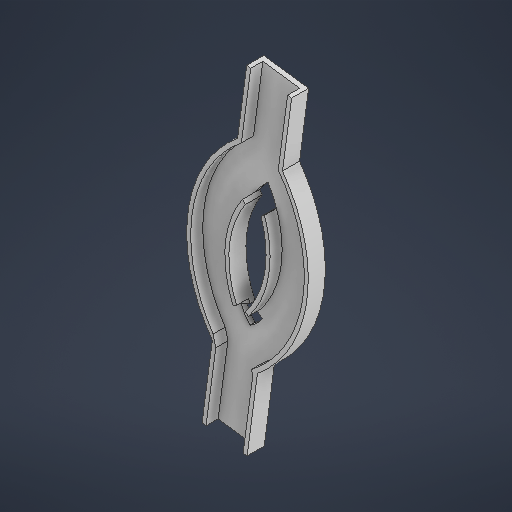
# Autodesk Inventor part: outside3
Saved by Autodesk Inventor 2026.2 (Build 302298000, 298)
## iProperties
Created: 2026-03-14
Part Number: outside3
Material: Generic
Document SubType Name: Modeling
Designer: danda
Density: 1 g/cm^3
Appearance: Default
Author: danda
Autodesk Inventor part; units mm, degrees
ref_plane "YZ Plane" through (0, 0, 0) normal (1, 0, 0) x (0, 1, 0)
ref_plane "XZ Plane" through (0, 0, 0) normal (0, 1, 0) x (-1, 0, 0)
ref_plane "XY Plane" through (0, 0, 0) normal (0, 0, 1) x (1, 0, 0)
sketch "Sketch1" plane through (0, 0, 0) normal (0, 0, 1) x (1, 0, 0)
  arc A0 (967.6192, 924.0732) -> (967.7873, 1075.2272) centre (902.2196, 999.723) ccw
  arc A1 (983.2683, 893.0126) -> (983.4428, 1106.3006) centre (902.2196, 999.723) ccw
  line L0 (965.7611, 927.7614) -> (985.0977, 889.3816)
  line L1 (966.6908, 925.9161) -> (1011.6908, 925.9161) construction
  arc A2 (985.0977, 889.3816) -> (985.2727, 1109.9327) centre (902.2196, 999.723) ccw
  line L2 (965.9281, 1071.5369) -> (985.2727, 1109.9327)
  arc A3 (965.7611, 927.7614) -> (965.9281, 1071.5369) centre (902.2196, 999.723) ccw
  line L3 (977.4986, 940.149) -> (980.6353, 937.6667)
  point P0 (0, 0)
  point P1 (983.9681, 893.1)
  point P2 (990.6031, 1100.4422)
  point P3 (968.1775, 1074.8866)
  dimension "d28" = 100
  dimension "d33" = 63.26
  dimension "d34" = 4
  dimension "d40" = 4
  dimension "d41" = 4
  constraints: 10 point on circle, 8 end point, 5 point on line, 4 centre point, 1 horizontal
  measures "d28" radius of A0
  measures "d33" angle of L0 L1
  measures "d34" radial gap between concentric circles of A1 A2
  measures "d40" radial gap between concentric circles of A0 A3
  measures "d41" distance of L3.start L3.end
extrude "Extrusion6" add sketch "Sketch1" along normal blind 5
extrude "Extrusion7" add sketch "Sketch1" along normal blind 17 contours L3 A3 L2 A0 | A1 L2 A2 L0
sketch "Sketch5" plane through (0, 0, 5) normal (0, 0, 1) x (1, 0, 0)
  arc A0 (965.7611, 927.7614) -> (977.4986, 940.149) centre (902.2196, 999.723) ccw projected
  line L0 (965.7611, 927.7614) -> (970.2605, 918.8308)
  line L1 (965.7611, 927.7614) -> (983.2683, 893.0126) projected
  line L2 (977.4986, 940.149) -> (985.1361, 933.6938)
  arc A1 (965.7611, 927.7614) -> (977.4986, 940.149) centre (902.2196, 999.723) ccw
  arc A2 (965.7611, 927.7614) -> (974.9009, 937.006) centre (902.2196, 999.723) ccw
  line L3 (974.9009, 937.006) -> (982.5384, 930.5509)
  arc A3 (970.2605, 918.8308) -> (982.5384, 930.5509) centre (950.8165, 951.4915) ccw
  point P0 (0, 0)
  dimension "d42" = 10
  dimension "d43" = 10
  dimension "d46" = 13
  dimension "d47" = 10
  constraints: 7 point on circle, 6 end point, 3 centre point, 1 concentric, 1 parallel, 1 point on line
  measures "d42" distance of L0.start L0.end
  measures "d43" distance of L2.start L2.end
  measures "d46" distance of L0.start L3.start
  measures "d47" distance of L3.start L3.end
extrude "Extrusion8" cut sketch "Sketch5" along normal through all both and the other way through all
sketch "Sketch6" plane through (0, 0, 5) normal (0, 0, 1) x (1, 0, 0)
  arc A0 (974.9009, 937.006) -> (965.9281, 1071.5369) centre (902.2196, 999.723) ccw projected
  arc A1 (985.0977, 889.3816) -> (985.2727, 1109.9327) centre (902.2196, 999.723) ccw projected
  line L0 (985.8441, 1046.8712) -> (1027.8759, 1046.8712) construction
  line L1 (985.2727, 1109.9327) -> (965.9281, 1071.5369) projected
  line L2 (965.9281, 1071.5369) -> (985.2727, 1109.9327)
  arc A2 (985.8441, 1046.8712) -> (965.9281, 1071.5369) centre (902.2196, 999.723) ccw
  arc A3 (1007.3627, 1089.1038) -> (985.2727, 1109.9327) centre (902.2196, 999.723) ccw
  line L3 (985.8441, 1046.8712) -> (1007.3627, 1089.1038)
  point P0 (0, 0)
  dimension "d51" = 63
  constraints: 6 end point, 6 point on circle, 2 centre point, 2 concentric, 1 collinear, 1 horizontal
  measures "d51" angle of L3 L0
extrude "Extrusion9" cut sketch "Sketch6" along normal through all both and the other way through all
sketch "Sketch7" plane through (0, 0, 5) normal (0, 0, 1) x (1, 0, 0)
  arc A0 (977.4782, 940.1232) -> (985.8441, 1046.8712) centre (902.2196, 999.723) ccw
  arc A1 (980.614, 937.6399) -> (988.005, 1051.1123) centre (902.2196, 999.723) ccw
  arc A2 (974.9009, 937.006) -> (985.8441, 1046.8712) centre (902.2196, 999.723) ccw projected
  line L0 (985.8441, 1046.8712) -> (988.005, 1051.1123)
  line L1 (985.8441, 1046.8712) -> (1007.3627, 1089.1038) projected
  line L2 (993.2753, 1030.1346) -> (996.6034, 1032.7639)
  point P0 (0, 0)
  dimension "d52" = 4
  constraints: 6 point on circle, 4 end point, 2 centre point, 1 point on line
  measures "d52" radial gap between concentric circles of A0 A1
extrude "Extrusion10" cut sketch "Sketch7" along normal through all both and the other way through all
sketch "Sketch8" plane through (0, 0, 17) normal (0, 0, 1) x (1, 0, 0)
  arc A0 (983.2683, 893.0126) -> (1005.3901, 1085.2324) centre (902.2196, 999.723) ccw projected
  arc A1 (1014.3006, 1073.1658) -> (1005.3901, 1085.2324) centre (902.2196, 999.723) ccw
  line L0 (988.005, 1051.1123) -> (1007.3627, 1089.1038) projected
  line L1 (1005.3901, 1085.2324) -> (1007.3627, 1089.1038)
  line L2 (1014.3006, 1073.1658) -> (1017.6463, 1075.3581)
  arc A2 (985.0977, 889.3816) -> (1007.3627, 1089.1038) centre (902.2196, 999.723) ccw projected
  arc A3 (1017.6463, 1075.3581) -> (1007.3627, 1089.1038) centre (902.2196, 999.723) ccw
  point P0 (0, 0)
  dimension "d55" = 15
  dimension "d56" = 4
  dimension "d57" = 138
  constraints: 6 point on circle, 4 end point, 2 centre point, 1 collinear
  measures "d55" distance of L1.start L2.start
  measures "d56" distance of L2.start L2.end
  measures "d57" radius of A3
extrude "Extrusion11" cut sketch "Sketch8" against normal blind 12
sketch "Sketch10" plane through (0, 0, 5) normal (0, 0, 1) x (1, 0, 0)
  line L0 (993.2753, 1030.1346) -> (996.6034, 1032.7639) projected
  arc A0 (996.6034, 1032.7639) -> (988.005, 1051.1123) centre (902.2196, 999.723) ccw projected
  line L1 (988.005, 1051.1123) -> (1007.3627, 1089.1038) projected
  arc A1 (1017.6463, 1075.3581) -> (1007.3627, 1089.1038) centre (902.2196, 999.723) ccw projected
  line L2 (1014.3006, 1073.1658) -> (1017.6463, 1075.3581) projected
  arc A2 (983.2683, 893.0126) -> (1014.3006, 1073.1658) centre (902.2196, 999.723) ccw projected
  line L3 (983.2683, 893.0126) -> (970.2605, 918.8308) projected
  arc A3 (970.2605, 918.8308) -> (982.5384, 930.5509) centre (950.8165, 951.4915) ccw projected
  line L4 (982.5384, 930.5509) -> (974.9009, 937.006) projected
  arc A4 (974.9009, 937.006) -> (977.4986, 940.149) centre (902.2196, 999.723) ccw projected
  arc A5 (977.4986, 940.149) -> (993.2753, 1030.1346) centre (902.2196, 999.723) ccw projected
  arc A6 (980.6353, 937.6667) -> (996.6034, 1032.7639) centre (902.2196, 999.723) ccw projected
  line L5 (977.4986, 940.149) -> (980.6353, 937.6667) projected
  arc A7 (985.0977, 889.3816) -> (1017.6463, 1075.3581) centre (902.2196, 999.723) ccw projected
  line L6 (985.0977, 889.3816) -> (983.2683, 893.0126) projected
  line L7 (970.2605, 918.8308) -> (988.005, 1051.1123)
  line L8 (977.3926, 1032.2651) -> (974.8751, 1035.6786)
  arc A8 (988.005, 1051.1123) -> (974.8751, 1035.6786) centre (1057.2145, 978.9317) ccw
  line L9 (988.005, 1051.1123) -> (979.3441, 1092.8623)
  arc A9 (979.3441, 1092.8623) -> (965.8014, 1082.3127) centre (1057.2145, 978.9317) ccw
  line L10 (968.4511, 1079.3162) -> (965.8014, 1082.3127)
  arc A10 (973.7155, 1083.7358) -> (945.5606, 904.8412) centre (1057.2145, 978.9317) ccw
  line L11 (950.9084, 897.3534) -> (970.2605, 918.8308)
  arc A11 (961.5054, 933.3723) -> (970.2605, 918.8308) centre (997.6246, 945.2125) ccw
  line L12 (961.5054, 933.3723) -> (970.5741, 937.5864)
  arc A12 (968.8965, 941.3029) -> (970.5741, 937.5864) centre (1057.2145, 978.9317) ccw
  arc A13 (977.3926, 1032.2651) -> (968.8965, 941.3029) centre (1057.2145, 978.9317) ccw
  arc A14 (974.8751, 1035.6786) -> (965.2166, 939.735) centre (1057.2145, 978.9317) ccw
  line L13 (968.8965, 941.3029) -> (965.2166, 939.735)
  arc A15 (965.8014, 1082.3127) -> (948.1868, 894.3329) centre (1057.2145, 978.9317) ccw
  line L14 (948.1868, 894.3329) -> (950.9084, 897.3534)
  line L15 (970.2605, 918.8308) -> (948.1868, 894.3329)
  line L16 (970.2605, 918.8308) -> (985.0977, 889.3816)
  line L17 (985.0977, 889.3816) -> (975.4208, 817.2429)
  line L18 (948.1868, 894.3329) -> (938.5099, 822.1942)
  line L19 (945.5606, 904.8412) -> (934.5454, 822.726)
  line L20 (934.5454, 822.726) -> (979.3853, 816.7111)
  line L21 (979.3853, 816.7111) -> (990.4004, 898.8263)
  line L22 (945.5606, 904.8412) -> (948.1868, 894.3329)
  line L23 (985.0977, 889.3816) -> (990.4004, 898.8263)
  line L24 (988.005, 1051.1123) -> (1007.3627, 1089.1038) projected
  line L25 (988.005, 1051.1123) -> (979.3441, 1092.8623)
  line L26 (988.005, 1051.1123) -> (1007.3627, 1089.1038)
  line L27 (978.9999, 1153.216) -> (1023.6004, 1147.2332)
  line L28 (970.2605, 918.8308) -> (988.005, 1051.1123)
  line L29 (978.9999, 1153.216) -> (969.9631, 1085.8484)
  line L30 (1023.6004, 1147.2332) -> (1014.5636, 1079.8656)
  line L31 (973.7155, 1083.7358) -> (982.9644, 1152.6842)
  line L32 (1019.6359, 1147.765) -> (1010.3871, 1078.8166)
  arc A16 (990.4004, 898.8263) -> (1010.3871, 1078.8166) centre (902.2196, 999.723) ccw
  point P0 (0, 0)
  point P1 (982.4326, 1148.7197)
  point P2 (1018.8217, 1141.6953)
  point P3 (980.2267, 1088.6079)
  point P4 (1005.3901, 1085.2324)
  point P5 (1011.1435, 1084.4555)
  point P6 (944.768, 898.933)
  point P7 (989.6079, 892.9181)
  point P8 (1001.3002, 1150.2246)
  point P9 (956.9654, 819.7185)
  dimension "d60" = 132.2815
  dimension "d61" = 4
  dimension "d62" = 4
  dimension "d64" = 45
  dimension "d65" = 22.5
  dimension "d66" = 4
  dimension "d74" = 100
  dimension "d75" = 100
  constraints: 50 end point, 22 point on circle, 21 symmetric about line, 9 centre point, 8 point on line, 5 parallel, 4 collinear, 2 midpoint, 2 perpendicular, 9 other
  measures "d60" vertical distance of L3.end L1.start
  measures "d61" distance between parallel lines of L18 L19
  measures "d62" distance between parallel lines of L17 L21
  measures "d64" distance of L27.start L27.end
  measures "d65" distance from line of L27.end L28
  measures "d66" distance between parallel lines of L29 L31
  measures "d74" distance from line of L1.start L27
  measures "d75" distance of point (956.965, 819.719) L3.end
extrude "Extrusion12" add sketch "Sketch10" against normal blind 5 contours L9 A9 L31 L27 L32 A1 L1 | A8 A14 L13 A12 L12 A11 L11 L14 L22 A10 L31 A9 L9 | L3 L6 L17 L20 L18 L14 L11
extrude "Extrusion13" add sketch "Sketch10" along normal blind 12 and the other way blind 5 contours L8 A13 L13 A14 | L32 L27 L30 A1 | A1 L2 A16 L32 | L31 A10 L10 A9 | A9 L29 L27 L31 | A7 L21 L20 L17 | L18 L20 L19 A15 | A15 L19 L22 | A15 L10 A10 L19
body "Solid2"
